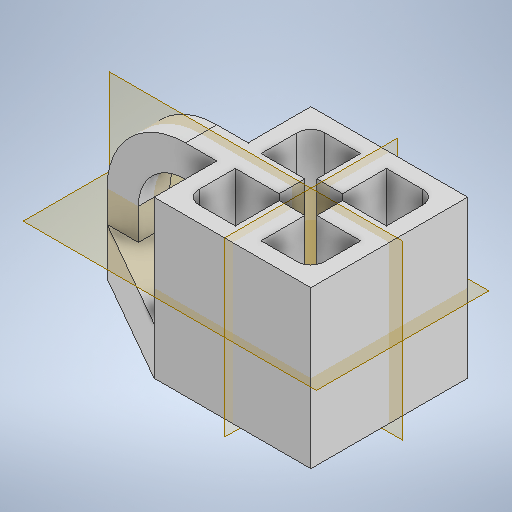
# Autodesk Inventor part: Pieza1AnclajePerfil
Saved by Autodesk Inventor 2025.2 (Build 292293000, 293)
## iProperties
Created: 2025-03-31
Part Number: Pieza1AnclajePerfil
Material: Genérico
Document SubType Name: Modeling
Designer: braug
Density: 1 g/cm^3
Appearance: Valor por defecto
Author: braug
Autodesk Inventor part; units mm, degrees
sketch "Boceto1" plane through (0, 0, 0) normal (0, 1, 0) x (-1, 0, 0)
  line L0 (25, -25) -> (-25, -25)
  line L1 (-25, -25) -> (25, -25)
  line L2 (25, -25) -> (25, 25)
  line L3 (25, 25) -> (-25, 25)
  line L4 (-25, 25) -> (-25, -25)
  line L5 (25, -25) -> (-25, 25) construction
  line L6 (-15.5, -20) -> (15.5, -20)
  line L7 (20, -15.5) -> (20, 15.5)
  line L8 (15.5, 20) -> (-15.5, 20)
  line L9 (-20, 15.5) -> (-20, -15.5)
  line L10 (-20, -20) -> (20, 20) construction
  line L11 (20, -20) -> (-20, 20) construction
  arc A0 (-20, -15.5) -> (-15.5, -20) centre (-15.7015, -15.7015) ccw
  line L12 (25, 25) -> (-12.318, -12.318) construction
  line L13 (-15.7015, -15.7015) -> (-25, -25) construction
  circle A1 centre (0, 0) radius 3.4
  line L14 (-4.5858, -6) -> (4.5858, -6)
  line L15 (6, -4.5858) -> (6, 4.5858)
  line L16 (4.5858, 6) -> (-4.5858, 6)
  line L17 (-6, 4.5858) -> (-6, -4.5858)
  line L18 (-5.4, -5.4) -> (5.4, 5.4) construction
  line L19 (5.4, -5.4) -> (-5.4, 5.4) construction
  line L20 (-4.5858, 6) -> (-9.9858, 11.4)
  line L21 (10.25, 23.8) -> (-10.25, 16.2) construction
  line L22 (-10.25, 23.8) -> (10.25, 16.2) construction
  line L23 (-9.9858, 20) -> (-9.9858, 11.4)
  line L24 (-11.2858, 12.7) -> (-11.2858, 20)
  line L25 (-20, 9.9858) -> (-11.4, 9.9858)
  line L26 (-12.7, 11.2858) -> (-20, 11.2858)
  line L27 (-6, 4.5858) -> (-11.4, 9.9858)
  arc A2 (-12.7, 11.2858) -> (-11.2858, 12.7) centre (-12.7, 12.7) ccw
  arc A3 (20, 15.5) -> (15.5, 20) centre (15.7015, 15.7015) ccw
  line L28 (0, 50.7962) -> (0, -27.7787) construction
  arc A4 (15.5, -20) -> (20, -15.5) centre (15.7015, -15.7015) ccw
  arc A5 (-15.5, 20) -> (-20, 15.5) centre (-15.7015, 15.7015) ccw
  line L29 (11.2858, -12.7) -> (11.2858, -20)
  line L30 (9.9858, -20) -> (9.9858, -11.4)
  line L31 (4.5858, -6) -> (9.9858, -11.4)
  line L32 (6, -4.5858) -> (11.4, -9.9858)
  line L33 (20, -9.9858) -> (11.4, -9.9858)
  arc A6 (12.7, -11.2858) -> (11.2858, -12.7) centre (12.7, -12.7) ccw
  line L34 (12.7, -11.2858) -> (20, -11.2858)
  line L35 (20, 9.9858) -> (11.4, 9.9858)
  line L36 (12.7, 11.2858) -> (20, 11.2858)
  line L37 (9.9858, 20) -> (9.9858, 11.4)
  line L38 (11.2858, 12.7) -> (11.2858, 20)
  arc A7 (11.2858, 12.7) -> (12.7, 11.2858) centre (12.7, 12.7) ccw
  line L39 (4.5858, 6) -> (9.9858, 11.4)
  line L40 (6, 4.5858) -> (11.4, 9.9858)
  line L41 (-6, -4.5858) -> (-11.4, -9.9858)
  line L42 (-4.5858, -6) -> (-9.9858, -11.4)
  line L43 (-9.9858, -20) -> (-9.9858, -11.4)
  line L44 (-11.2858, -12.7) -> (-11.2858, -20)
  arc A8 (-11.2858, -12.7) -> (-12.7, -11.2858) centre (-12.7, -12.7) ccw
  line L45 (-12.7, -11.2858) -> (-20, -11.2858)
  line L46 (-20, -9.9858) -> (-11.4, -9.9858)
  line L47 (11.2858, 12.7) -> (11.2858, 18.2358)
  line L48 (11.2858, 18.2358) -> (15.7015, 18.2358)
  line L49 (18.2358, 15.7015) -> (18.2358, 11.2858)
  line L50 (18.2358, 11.2858) -> (12.7, 11.2858)
  line L51 (-18.2358, -11.2858) -> (-18.2358, -18.2358)
  line L52 (-18.2358, -18.2358) -> (-11.2858, -18.2358)
  line L53 (-11.2858, 18.2358) -> (-18.2358, 18.2358)
  line L54 (-18.2358, 18.2358) -> (-18.2358, 11.2858)
  line L55 (18.2358, -18.2358) -> (11.2858, -18.2358)
  line L56 (18.2358, -11.2858) -> (18.2358, -18.2358)
  arc A9 (18.2358, 15.7015) -> (15.7015, 18.2358) centre (15.7015, 15.7015) ccw
  line L57 (4.1, 6.9873) -> (4.1, 20)
  line L58 (4.1, 20) -> (-4.1, 20)
  line L59 (-4.1, 20) -> (-4.1, 6.9873)
  line L60 (-4.1, 20) -> (-4.1, 6)
  line L61 (4.1, 20) -> (4.1, 6)
  line L62 (-20, 4.1) -> (-6, 4.1)
  line L63 (-20, -4.1) -> (-6, -4.1)
  line L64 (20, -4.1) -> (6, -4.1)
  line L65 (20, 4.1) -> (6, 4.1)
  line L66 (4.1, -20) -> (4.1, -6)
  line L67 (-4.1, -20) -> (-4.1, -6)
  point P0 (0, 0)
  point P1 (0, -25)
  point P2 (0, 20)
  point P3 (18.2358, 18.2358)
  point P4 (0, 13.4937)
  point P5 (6.9873, -4.1)
  point P6 (20, -4.1)
  point P7 (4.1, -6)
  point P8 (-4.1, -20)
  point P9 (-6, -4.1)
  point P10 (-6, 4.1)
  point P11 (6, 4.1)
  dimension "d0" = 50
  dimension "d1" = 50
  dimension "d2" = 40
  dimension "d3" = 40
  dimension "d4" = 6.8
  dimension "d5" = 1
  dimension "d6" = 20.5
  dimension "d7" = 1.3
  dimension "d8" = 6.95
  dimension "d9" = 6.95
  dimension "d10" = 14
  dimension "d11" = 14
  dimension "d12" = 40
  dimension "d13" = 8.2
  constraints: 136 end point, 67 symmetric about line, 18 point on circle, 12 parallel, 12 point on line, 10 centre point, 7 midpoint, 6 perpendicular, 3 coincident, 3 horizontal, 3 vertical, 1 tangent, 6 other
  measures "d0" distance of L3.end L12.start
  measures "d1" distance of L12.start L1.end
  measures "d2" distance of L11.end L10.end
  measures "d3" distance of L10.end L11.start
  measures "d4" diameter of A1
  measures "d5" distance between parallel lines of L11 L20
  measures "d6" distance of L22.end L21.end
  measures "d7" distance between parallel lines of L24 L23
  measures "d8" distance of L48.start point (18.236, 18.236)
  measures "d9" distance between parallel lines of L50 L48
  measures "d10" distance between parallel lines of L8 L16
  measures "d11" distance between parallel lines of L6 L14
  measures "d12" distance between parallel lines of L6 L8
  measures "d13" distance of L60.start L57.end
extrude "Extrusión1" add sketch "Boceto1" along normal mid plane 50 contours L0 L4 L3 L2 | L67 L14 L66 L6 | L9 L62 L17 L63 | L64 L15 L65 L7 | L8 L57 L61 L16 L60 L59
sketch "Boceto2" plane through (0, 0, 0) normal (0, 0, 1) x (1, 0, 0)
  point P0 (0, 0)
sketch "Boceto3" plane through (0, 0, 0) normal (0, 0, 1) x (1, 0, 0)
  line L0 (-60, -10) -> (-10, -10)
  line L1 (-45, 0) -> (-45, -10)
  arc A0 (-35, 10) -> (-45, 0) centre (-35, 0) ccw
  arc A1 (-35, 15) -> (-50, 0) centre (-35, 0) ccw
  line L2 (-50, 0) -> (-50, -10)
  arc A2 (-35, 25) -> (-60, 0) centre (-35, 0) ccw
  line L3 (-60, 0) -> (-60, -10)
  line L4 (-60, -10) -> (-35, -10)
  circle A3 centre (-35, 0) radius 5.2
  line L5 (-35, 10) -> (-25, 10)
  line L6 (-25, 10) -> (-25, 11.1803)
  line L7 (-25, 15) -> (-35, 15)
  line L8 (-35, 25) -> (-25, 25)
  line L9 (-25, 25) -> (-25, 15)
  line L10 (-25, 10) -> (-25, -10)
  line L11 (-25, -10) -> (-35, -10)
  line L12 (-25, -25) -> (-25, 25) projected
  point P0 (0, 0)
  point P1 (39.4507, -29.1043)
  dimension "d16" = 20
  dimension "d17" = 25
  dimension "d18" = 10
  dimension "d19" = 10
  dimension "d20" = 10.4
  dimension "d21" = 10
  dimension "d22" = 35
  constraints: 24 end point, 7 point on circle, 5 point on line, 4 centre point, 3 coincident, 3 perpendicular, 3 tangent, 2 collinear, 1 horizontal, 1 midpoint, 1 parallel
  measures "d16" distance of L5.start L4.end
  measures "d17" distance of L7.end L4.end
  measures "d18" distance of L3.start L0.start
  measures "d19" distance of L4.end A2.centre
  measures "d20" diameter of A3
  measures "d21" distance of L5.start L6.start
  measures "d22" distance of L10.end L8.end
extrude "Extrusión2" add sketch "Boceto3" along normal mid plane 10 contours L3 A2 L8 L9 L7 A1 L2 L0 | L1 A0 L5 L10 L0
sketch "Boceto4" plane through (-45, -10, 5) normal (0, -1, 0) x (1, 0, 0)
  line L0 (20, 20) -> (70, 20) projected
  line L1 (-15, 0) -> (-5, 0) projected
  line L2 (20, 20) -> (-15, 0)
  line L3 (-15, 0) -> (-15, -10)
  line L4 (20, -30) -> (70, -30) projected
  line L5 (-15, -10) -> (20, -30)
  line L6 (20, -30) -> (20, 20)
  line L7 (-5, -10) -> (-15, -10) projected
  point P0 (45, -5)
  constraints: 8 end point, 2 perpendicular
extrude "Extrusión3" add sketch "Boceto4" along normal up to surface (15 mm away)
